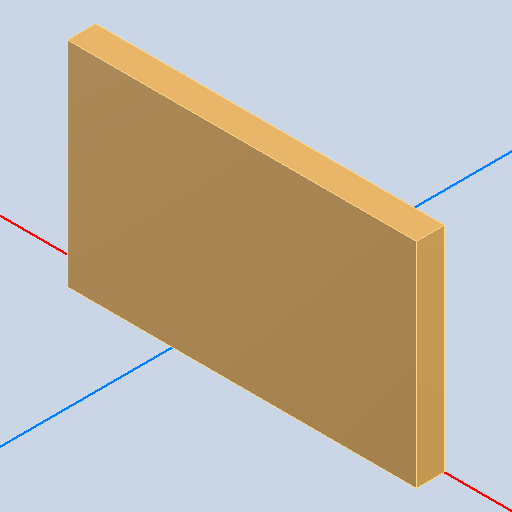
# Autodesk Inventor part: J2_SCREWTERMINAL-5MM-2
Saved by Autodesk Inventor 2022 (Build 260153000, 153)
## iProperties
Created: 2023-03-06
Part Number: J2_SCREWTERMINAL-5MM-2
Material: Типовые
Document SubType Name: Modeling
Designer: Иван Петров
Density: 1 g/cm^3
Appearance: SCREWTERMINAL-5MM-2, J2_SCREWTERMINAL-5MM-2
Author: Иван Петров
Autodesk Inventor part; units mm, degrees
ref_plane "YZ Plane" through (0, 0, 0) normal (1, 0, 0) x (0, 1, 0)
ref_plane "XZ Plane" through (0, 0, 0) normal (0, 1, 0) x (-1, 0, 0)
ref_plane "XY Plane" through (0, 0, 0) normal (0, 0, 1) x (1, 0, 0)
sketch "SCREWTERMINAL-5MM-2, J2_SCREWTERMINAL-5MM-2_6" plane through (0, 0, 0) normal (0, 0, 1) x (1, 0, 0)
  line L0 (-3.7, 4.3016) -> (8.7, 4.3016)
  line L1 (8.7, 4.3016) -> (8.7, -3.3)
  line L2 (8.7, -3.3) -> (-3.7, -3.3)
  line L3 (-3.7, -3.3) -> (-3.7, 4.3016)
  constraints: 8 end point
extrude "Выдавливание1" add sketch "SCREWTERMINAL-5MM-2, J2_SCREWTERMINAL-5MM-2_6" along normal blind 1
